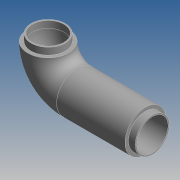
# Autodesk Inventor part: P008_CanonBout
Saved by Autodesk Inventor 2020 (Build 240168000, 168)
## iProperties
Created: 2021-10-15
Part Number: P008_CanonBout
Material: Générique
Document SubType Name: Modeling
Designer: gabri
Density: 1 g/cm^3
Appearance: Par défaut
Author: gabri
Autodesk Inventor part; units mm, degrees
ref_plane "YZ Plane" through (0, 0, 0) normal (1, 0, 0) x (0, 1, 0)
ref_plane "XZ Plane" through (0, 0, 0) normal (0, 1, 0) x (-1, 0, 0)
ref_plane "XY Plane" through (0, 0, 0) normal (0, 0, 1) x (1, 0, 0)
sketch "Esquisse9" plane through (0, 0, 0) normal (0, 1, 0) x (-1, 0, 0)
  line L0 (0, 0) -> (100, 0)
  arc A0 (100, 0) -> (142.4264, 42.4264) centre (100, 42.4264) ccw
  line L1 (181.4558, 0) -> (-30.2426, 0) construction
  dimension "d20" = 100
  dimension "d21" = 60
  dimension "d37" = 42.4264
  constraints: 2 end point, 2 point on circle, 1 centre point, 1 horizontal, 1 tangent
  measures "d20" distance of L0.start L0.end
  measures "d21" distance of L0.end A0.end
  measures "d37" distance from line of L1 A0.centre
sketch "Esquisse10" plane through (0, 0, 0) normal (1, 0, 0) x (0, 1, 0)
  circle A0 centre (0, 0) radius 30
  circle A1 centre (0, 0) radius 23
  dimension "d22" = 60
  dimension "d23" = 46
  constraints: 2 centre point, 2 coincident
  measures "d22" diameter of A0
  measures "d23" diameter of A1
sweep "Balayage2" add profiles "Esquisse10" path "Esquisse9"
sketch "Esquisse11" plane through (0, 0, 0) normal (1, 0, 0) x (0, 0, -1)
  circle A0 centre (0, 0) radius 23 construction
  circle A1 centre (0, 0) radius 30 construction
  circle A2 centre (0, 0) radius 23
  circle A3 centre (0, 0) radius 25
  dimension "d26" = 50
  constraints: 2 centre point, 2 coincident, 1 concentric
  measures "d26" diameter of A3
extrude "Extrusion4" add sketch "Esquisse11" along normal blind 10
sketch "Esquisse14" plane through (-142.4264, 0, 42.4264) normal (0, 0, 1) x (1, 0, 0)
  circle A0 centre (0, 0) radius 23 construction
  circle A1 centre (0, 0) radius 30 construction
  circle A2 centre (0, 0) radius 23
  circle A3 centre (0, 0) radius 25
  point P0 (142.4264, 0)
  dimension "d38" = 50
  constraints: 2 centre point, 2 coincident, 1 concentric
  measures "d38" diameter of A3
extrude "Extrusion5" add sketch "Esquisse14" along normal blind 10
